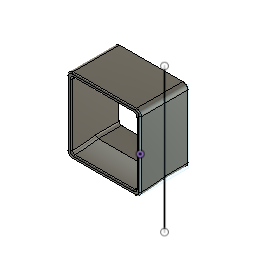
TAP-DIVERGE-REDUCED (Autodesk Fusion 360 design; units mm, degrees)
Autodesk Fusion 360 part; units mm, degrees
note: some values were not read from the file. Chosen so that the rebuilt part matches the saved one: which pieces of a blend or face edit are solid.
sketch "Sketch1" plane through (0, 0, 0) normal (0, 1, 0) x (1, 0, 0)
  line L0 (15, -15) -> (-15, -15)
  line L1 (-15, -15) -> (-15, 15)
  line L2 (-15, 15) -> (15, 15)
  line L3 (15, 15) -> (15, -15)
  line L4 (15, -15) -> (-15, 15) construction
  line L5 (-15, -15) -> (15, 15) construction
  dimension "d1" = 30
  dimension "d2" = 30
  constraint horizontal L0
  constraint perpendicular L0 L1
  constraint parallel L0 L2
  constraint parallel L1 L3
  constraint coincident L4 origin
  constraint coincident L5 origin
  measures "d1" distance of L1.end L2.end
  measures "d2" distance of L0.end L1.end
extrude "Extrude1" add sketch "Sketch1" along normal blind 20
sketch "Sketch2" plane through (0, 0, 0) normal (0, -1, 0) x (1, 0, 0)
  line L0 (-15, -15) -> (15, -15)
  line L1 (15, -15) -> (15, 15)
  line L2 (15, 15) -> (-15, 15)
  line L3 (-15, 15) -> (-15, -15)
  line L4 (13.25, -13.25) -> (-13.25, -13.25)
  line L5 (-13.25, -13.25) -> (-13.25, 13.25)
  line L6 (-13.25, 13.25) -> (13.25, 13.25)
  line L7 (13.25, 13.25) -> (13.25, -13.25)
  line L8 (13.25, -13.25) -> (-13.25, 13.25) construction
  line L9 (-13.25, -13.25) -> (13.25, 13.25) construction
  dimension "d5" = 26.5
  dimension "d6" = 26.5
  constraint horizontal L4
  constraint perpendicular L4 L5
  constraint parallel L4 L6
  constraint parallel L5 L7
  constraint coincident L8 origin
  constraint coincident L9 origin
  measures "d5" distance of L5.end L6.end
  measures "d6" distance of L4.end L5.end
extrude "Extrude2" cut sketch "Sketch2" against normal through all contours L4 L5 L6 L7
sketch "Sketch3" plane through (15, 0, 0) normal (1, 0, 0) x (0, 1, 0)
  line L0 (0, 15) -> (0, -15)
  line L1 (0, -15) -> (20, -15)
  line L2 (20, -15) -> (20, 15)
  line L3 (20, 15) -> (0, 15)
  line L4 (10, 26.2783) -> (10, -32.7983)
  dimension "d18" = 10
  constraint vertical L4
  measures "d18" distance of origin L4
sketch "Sketch4" plane through (15, 0, 0) normal (1, 0, 0) x (0, 1, 0)
sketch "Sketch5" plane through (15, 0, 0) normal (1, 0, 0) x (0, 1, 0)
  arc A0 (0, -15.8842) -> (10.4099, -15) centre (-0.3235, 49.6471) ccw
  line L0 (0, -15.8842) -> (0, -15)
  line L1 (0, -15) -> (10.4099, -15)
  constraint vertical L0
  constraint perpendicular L0 L1
extrude "Extrude3" add sketch "Sketch5" against normal blind 30
sketch "Sketch6" plane through (0, 0, 0) normal (0, -1, 0) x (1, 0, 0)
  line L0 (13.25, 13.25) -> (13.25, -13.25)
  line L1 (13.25, -13.25) -> (-13.25, -13.25)
  line L2 (-13.25, -13.25) -> (-13.25, 13.25)
  line L3 (-13.25, 13.25) -> (13.25, 13.25)
  line L4 (15, -15.8842) -> (15, 15)
  line L5 (15, 15) -> (-15, 15)
  line L6 (-15, 15) -> (-15, -15.8842)
  line L7 (-15, -15.8842) -> (15, -15.8842)
  line L8 (-13.25, -13.25) -> (-13.25, -14.1342)
  line L9 (-13.25, -14.1342) -> (13.245, -14.1342)
  line L10 (13.245, -14.1342) -> (13.25, -13.25)
  dimension "d10" = 1.95
  dimension "d11" = 1.75
  constraint coincident L1.end L2.start
  constraint perpendicular L1 L8
  constraint perpendicular L2 L9
  constraint coincident L0.end L1.start
  measures "d11" distance of L7 L9
sweep "Sweep1" cut profiles "Sketch6" along 1 edges at (15, 5.2226, -15.6499) section 1 contours L1 L8 L9 L10
fillet "Fillet1" radius 2 6 edges at (-15, 10, 15) (15, 10, 15) (-15, 5.2226, -15.6499) (15, 15.205, -15) (15, 5.2226, -15.6499) (-15, 15.205, -15)
fillet "Fillet2" radius 1 6 edges at (-13.25, 10, 13.25) (13.25, 10, 13.25) (-13.25, 15.0641, -13.25) (13.25, 10, -13.25) (-13.25, 5.0831, -13.9054) (13.245, 5.0831, -13.9054)
fillet "Fillet3" radius 0.5 16 edges at (-14.4142, 0, 14.4142) (-15, 0, -0.4421) (-14.4142, 0, -15.2984) (0, 0, -15.8842) (14.4142, 0, -15.2984) (15, 0, -0.4421) (14.4142, 0, 14.4142) (0, 0, 15) (12.9214, 0, -13.8814) (0.0034, 0, -14.1342) (-12.9571, 0, -13.8413) (-13.25, 0, -0.4421) (-12.9571, 0, 12.9571) (0, 0, 13.25) (12.9571, 0, 12.9571) (13.25, 0, -0.5)
fillet "Fillet4" radius 0.5 16 edges at (14.4142, 20, 14.4142) (15, 20, 0) (14.4142, 20, -14.4142) (0, 20, -15) (-14.4142, 20, -14.4142) (-15, 20, 0) (-14.4142, 20, 14.4142) (0, 20, 15) (-12.9571, 20, 12.9571) (-13.25, 20, 0) (-12.9571, 20, -12.9571) (0, 20, -13.25) (12.9571, 20, -12.9571) (13.25, 20, 0) (12.9571, 20, 12.9571) (0, 20, 13.25)
